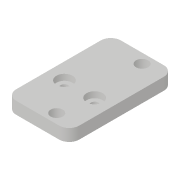
# Autodesk Inventor part: SwitchHolderTNutRight
Saved by Autodesk Inventor 2018 (Build 220112000, 112)
## iProperties
Created: 2018-12-20
Part Number: SwitchHolderTNutRight
Material: Generic
Document SubType Name: Modeling
Designer: ball
Density: 1 g/cm^3
Appearance: Default
Author: ball
Autodesk Inventor part; units mm, degrees
ref_plane "YZ Plane" through (0, 0, 0) normal (1, 0, 0) x (0, 1, 0)
ref_plane "XZ Plane" through (0, 0, 0) normal (0, 1, 0) x (-1, 0, 0)
ref_plane "XY Plane" through (0, 0, 0) normal (0, 0, 1) x (1, 0, 0)
sketch "Sketch1" plane through (0, 0, 0) normal (0, 1, 0) x (-1, 0, 0)
  line L0 (0, 0) -> (-19.8882, 0)
  line L1 (-19.8882, 0) -> (-19.8882, -33.02)
  line L2 (-19.8882, -33.02) -> (0, -33.02)
  line L3 (0, -33.02) -> (0, 0)
  circle A0 centre (-12.9032, -3.048) radius 1.905
  circle A1 centre (-12.9032, -29.972) radius 1.905
  dimension "d0" = 19.8882
  dimension "d1" = 33.02
  dimension "d2" = 3.81
  dimension "d3" = 3.048
  dimension "d4" = 6.985
  dimension "d5" = 3.81
  dimension "d6" = 3.048
  constraints: 8 end point, 2 centre point, 2 parallel, 1 horizontal, 1 perpendicular
  measures "d0" distance of L2.end L1.end
  measures "d1" distance of L1.end L0.end
  measures "d2" diameter of A0
  measures "d3" distance from line of L0 A0.centre
  measures "d4" distance from line of L1 A0.centre
  measures "d5" diameter of A1
  measures "d6" distance from line of L2 A1.centre
extrude "Extrusion1" add sketch "Sketch1" along normal blind 3.81
sketch "Sketch2" plane through (0, 3.81, 0) normal (0, 1, 0) x (1, 0, 0)
  circle A0 centre (5.1816, 13.208) radius 1.1938
  circle A1 centre (14.7066, 13.208) radius 1.1938
  circle A2 centre (12.9032, 3.048) radius 1.905 projected
  point P0 (0, 0)
  dimension "d9" = 2.3876
  dimension "d10" = 2.3876
  dimension "d11" = 7.7216
  dimension "d12" = 1.8034
  dimension "d13" = 10.16
  dimension "d14" = 10.16
  constraints: 2 centre point
  measures "d9" diameter of A0
  measures "d10" diameter of A1
  measures "d11" horizontal distance of A2.centre A0.centre
  measures "d12" horizontal distance of A2.centre A1.centre
  measures "d13" vertical distance of A2.centre A1.centre
  measures "d14" vertical distance of A2.centre A0.centre
hole "Hole1" at (5.1816, 3.81, -13.208) at (14.7066, 3.81, -13.208) direction (0, -1, 0) diameter 2.3876 end through all counterbore diameter 5.08 counterbore depth 1.905
fillet "Fillet1" radius 3.175 4 edges at (19.8882, 1.905, -33.02) (0, 1.905, -33.02) (19.8882, 1.905, 0) (0, 1.905, 0)
body "Solid1"
